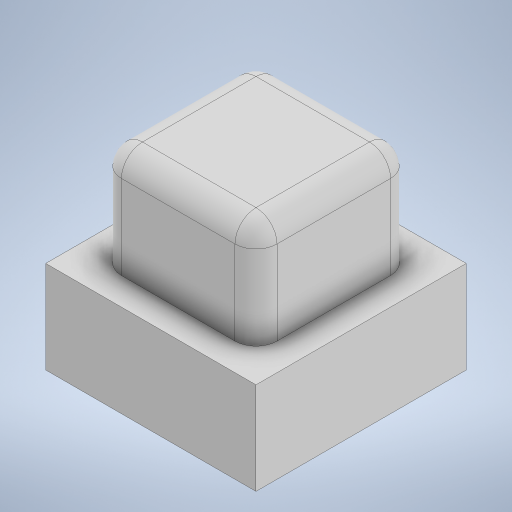
# Autodesk Inventor part: button
Saved by Autodesk Inventor 2024 (Build 280153000, 153)
## iProperties
Created: 2023-11-17
Part Number: button
Material: Générique
Document SubType Name: Modeling
Designer: digiacom
Density: 1 g/cm^3
Appearance: Par défaut
Author: digiacom
Autodesk Inventor part; units mm, degrees
ref_plane "YZ Plane" through (0, 0, 0) normal (1, 0, 0) x (0, 1, 0)
ref_plane "XZ Plane" through (0, 0, 0) normal (0, 1, 0) x (-1, 0, 0)
ref_plane "XY Plane" through (0, 0, 0) normal (0, 0, 1) x (1, 0, 0)
sketch "Esquisse6" plane through (0, 0, 0) normal (0, 1, 0) x (-1, 0, 0)
  line L0 (-6.8895, 5.7651) -> (-1.8895, 5.7651)
  line L1 (-1.8895, 5.7651) -> (-1.8895, 0.7651)
  line L2 (-1.8895, 0.7651) -> (-6.8895, 0.7651)
  line L3 (-6.8895, 0.7651) -> (-6.8895, 5.7651)
  point P0 (0, 0)
  dimension "d12" = 5
  dimension "d13" = 5
  constraints: 8 end point, 2 parallel, 1 horizontal, 1 perpendicular
  measures "d12" distance of L1.end L2.end
  measures "d13" distance of L0.end L1.end
extrude "Extrusion5" add sketch "Esquisse6" along normal blind 2.195
sketch "Esquisse7" plane through (0, 0, 0) normal (0, -1, 0) x (1, 0, 0)
  line L0 (6.8895, 5.7651) -> (6.8895, 0.7651) projected
  line L1 (6.8895, 0.7651) -> (1.8895, 0.7651) projected
  circle A0 centre (4.3895, 3.2651) radius 1.85
  point P0 (0, 0)
  dimension "d19" = 3.7
  constraints: 1 centre point
  measures "d19" diameter of A0
extrude "Extrusion6" cut sketch "Esquisse7" against normal blind 1.195
sketch "Esquisse8" plane through (0, 2.195, 0) normal (0, 1, 0) x (1, 0, 0)
  line L0 (2.5395, -5.1151) -> (6.2395, -5.1151)
  line L1 (6.2395, -5.1151) -> (6.2395, -1.4151)
  line L2 (6.2395, -1.4151) -> (2.5395, -1.4151)
  line L3 (2.5395, -1.4151) -> (2.5395, -5.1151)
  point P0 (0, 0)
  constraints: 8 end point, 2 parallel, 1 horizontal, 1 perpendicular
extrude "Extrusion7" add sketch "Esquisse8" along normal blind 2.5
fillet "Congé2" radius 0.5 4 edges at (4.3895, 4.695, 5.1151) (6.2395, 4.695, 3.2651) (4.3895, 4.695, 1.4151) (2.5395, 4.695, 3.2651)
fillet "Congé3" radius 0.5 8 edges at (2.686, 4.5486, 1.5615) (2.5395, 3.195, 1.4151) (2.686, 4.5486, 4.9686) (2.5395, 3.195, 5.1151) (6.0931, 4.5486, 4.9686) (6.2395, 3.195, 5.1151) (6.0931, 4.5486, 1.5615) (6.2395, 3.195, 1.4151)
